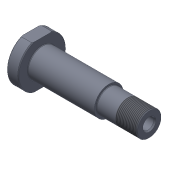
# Autodesk Inventor part: NA-45-h-Crown-277
Saved by Autodesk Inventor 2020.2 (Build 242310000, 310)
## iProperties
Created: 2020-04-21
Part Number: NA-45-h-Crown-277
Material: 16 341
Description: SROUBOVY CEP
Document SubType Name: Modeling
Designer: Jurek
Density: 7.85 g/cm^3
Appearance: RAL 7040 Window Grey(4)
Mass: 182.318 g
Surface Area: 87.1815 cm^2
Volume: 23.2253 cm^3
User Status: Rychlá změna
Checked By: Pippal
Category: B
Hmotnost (kg): 0,18
Rozmer_A: 33
Rozmer_B: 0
Rozmer_C: 0
Rozmer_D: 82
Rada vyrobku: 4100
Prumer nadobky: 45
Cislo artiklu: 4451101379
Jednotka: ks
Cisty rozmer: =Ø<Rozmer_A> - <Rozmer_D>
Predpona: Ø
Stroj na lince: Stahovací lis
RAZ Poznamka 1: ISO 2768-mH
RAZ Poznamka 2: NEOZNAČENÉ HRANY OJEHLIT
DXF: Ne
QAD_code: M
Rizeni davek: L
Author: Jurek
Revision Number: 00
Autodesk Inventor part; units mm, degrees
ref_plane "YZ Plane" through (0, 0, 0) normal (1, 0, 0) x (0, 1, 0)
ref_plane "XZ Plane" through (0, 0, 0) normal (0, 1, 0) x (-1, 0, 0)
ref_plane "XY Plane" through (0, 0, 0) normal (0, 0, 1) x (1, 0, 0)
sketch "Náčrt1" plane through (0, 0, 0) normal (0, 0, 1) x (1, 0, 0)
  line L0 (0, 0) -> (19.1477, 0)
  line L1 (0, 4) -> (0, 16.5)
  line L2 (0, 16.5) -> (8, 16.5)
  line L3 (8, 16.5) -> (8, 10.385)
  line L4 (8.4, 9.985) -> (54, 9.985)
  line L5 (54, 9.985) -> (54, 8.9)
  line L6 (54.4, 8.5) -> (82, 8.5)
  line L7 (82, 8.5) -> (82, 4)
  line L8 (82, 4) -> (0, 4)
  arc A0 (8, 10.385) -> (8.4, 9.985) centre (8.4, 10.385) ccw
  arc A1 (54, 8.9) -> (54.4, 8.5) centre (54.4, 8.9) ccw
  point P0 (54, 8.5)
  point P1 (8, 9.985)
  dimension "d0" = 33
  dimension "d1" = 82
  dimension "d2" = 28
  dimension "d5" = 17
  dimension "d6" = 8
  dimension "d7" = 19.97
  dimension "d8" = 74
  dimension "d39" = 8
  dimension "d40" = 46
  dimension "d41" = 0.4
  dimension "d42" = 0.4
  constraints: 18 end point, 6 parallel, 5 point on line, 4 point on circle, 4 tangent, 2 centre point, 2 perpendicular, 1 horizontal
  measures "d0" diameter of L2 L0
  measures "d1" distance between parallel lines of L7 L1
  measures "d2" distance between parallel lines of L7 L5
  measures "d5" diameter of L6 L0
  measures "d6" diameter of L8 L0
  measures "d7" diameter of L4 L0
  measures "d8" distance between parallel lines of L3 L7
  measures "d39" distance of L1.end L2.end
  measures "d40" distance between parallel lines of L5 L3
  measures "d41" radius of A0
  measures "d42" radius of A1
revolve "Rotace1" add sketch "Náčrt1" angle 360 about axis through (0, 0, 0) along (1, 0, 0)
thread "Závit1" size "M17x1" class "6g" standard "ANSI Metric M Profile" length 15
chamfer "Zkosení1" distance 0.5 angle 45 1 edges at (0, -16.5, 0)
chamfer "Zkosení2" distance 0.5 angle 45 1 edges at (8, -16.5, 0)
chamfer "Zkosení3" distance 1 angle 30 1 edges at (0, -4, 0) measured on face at (54.6667, 3.987, -0.3219)
chamfer "Zkosení4" distance 1 angle 30 1 edges at (82, -4, 0) measured on face at (55, 3.987, -0.3219)
chamfer "Zkosení5" distance 0.5 angle 45 1 edges at (82, -8.5, 0)
sketch "Náčrt2" plane through (0, 0, 0) normal (-1, 0, 0) x (0, 0, 1)
  line L0 (-15, 6.8739) -> (-17.8524, 6.8739)
  line L1 (-17.8524, 6.8739) -> (-17.8524, -6.8739)
  line L2 (-17.8524, -6.8739) -> (-15, -6.8739)
  line L3 (-15, -6.8739) -> (-15, 6.8739)
  line L4 (19.6486, 6.8739) -> (15, 6.8739)
  line L5 (15, 6.8739) -> (15, -6.8739)
  line L6 (15, -6.8739) -> (19.6486, -6.8739)
  line L7 (19.6486, -6.8739) -> (19.6486, 6.8739)
  line L8 (0, 0) -> (0, -4.618) construction
  circle A0 centre (0, 0) radius 16.5 construction
  dimension "d29" = 30
  constraints: 18 end point, 5 parallel, 2 horizontal, 2 perpendicular, 2 point on circle, 2 point on line, 1 other
  measures "d29" distance between parallel lines of L5 L3
extrude "Vysunutí1" cut sketch "Náčrt2" against normal through all
equation "\"Rozmer_A\" = d0"
equation "\"Rozmer_B\" = 0"
equation "\"Rozmer_C\" = 0"
equation "\"Rozmer_D\" = d1"
